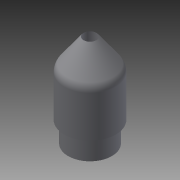
# Autodesk Inventor part: tipthick1024
Saved by Autodesk Inventor 2014 SP1 (Build 180222100, 222)
## iProperties
Created: 2014-05-29
Part Number: tipthick1024
Material: Generic
Document SubType Name: Modeling
Designer: lukeiseman
Density: 1 g/cm^3
Appearance: Default
Author: lukeiseman
Autodesk Inventor part; units mm, degrees
ref_plane "YZ Plane" through (0, 0, 0) normal (1, 0, 0) x (0, 1, 0)
ref_plane "XZ Plane" through (0, 0, 0) normal (0, 1, 0) x (-1, 0, 0)
ref_plane "XY Plane" through (0, 0, 0) normal (0, 0, 1) x (1, 0, 0)
sketch "Sketch1" plane through (0, 0, 0) normal (0, 0, 1) x (1, 0, 0)
  line L0 (0, 0) -> (6.35, 0)
  line L1 (6.35, 0) -> (6.35, 10.16)
  line L2 (0, 17.78) -> (1.5875, 17.78)
  line L3 (1.5875, 17.78) -> (5.7488, 12.0191)
  arc A0 (6.35, 10.16) -> (5.7488, 12.0191) centre (3.175, 10.16) ccw
  line L4 (0, 0) -> (3.175, 0)
  line L5 (1.5875, 17.78) -> (1.5875, 0)
  line L6 (6.35, 0) -> (1.5875, 0)
  line L7 (0, -3.556) -> (0, 21.336) projected
  dimension "d0" = 6.35
  dimension "d3" = 1.5875
  dimension "d4" = 3.175
  dimension "d9" = 10.16
  dimension "d10" = 17.78
  constraints: 14 end point, 2 midpoint, 2 perpendicular, 2 point on circle, 2 tangent, 1 centre point, 1 horizontal
  measures "d0" distance of L0.start L0.end
  measures "d3" distance of L2.start L2.end
  measures "d4" radius of A0
  measures "d9" distance of L0.end L1.end
  measures "d10" distance of L2.end L5.end
revolve "Revolution1" add sketch "Sketch1" angle 360 about axis through (0, -10, 0) along (0, 1, 0) contours L5 L3 A0 L1 L0
sketch "Sketch2" plane through (0, 0, 0) normal (0, -1, 0) x (1, 0, 0)
  circle A0 centre (0, 0) radius 1.5875 projected
  circle A1 centre (0, 0) radius 1.5875
  circle A2 centre (0, 0) radius 5.3975
  dimension "d6" = 10.795
  constraints: 2 centre point, 2 coincident, 1 concentric
  measures "d6" diameter of A2
extrude "Extrusion1" add sketch "Sketch2" along normal blind 5.08
body "Solid1"
